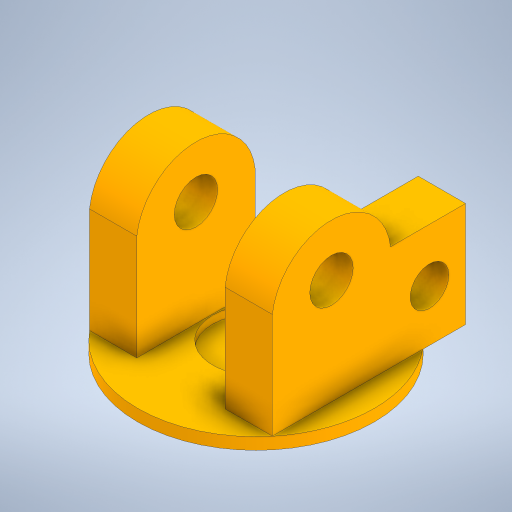
# Autodesk Inventor part: base2
Saved by Autodesk Inventor 2024 (Build 280153000, 153)
## iProperties
Created: 2024-04-28
Part Number: base2
Material: Generic
Document SubType Name: Modeling
Designer: samue
Density: 1 g/cm^3
Appearance: Default
Author: samue
## iProperties of the stored document base2_3DPrint.ipt
Created: 2024-04-28
Part Number: base2_3DPrint
Material: Generic
Document SubType Name: Modeling
Designer: samue
Density: 1 g/cm^3
Appearance: Default
Author: samue
Autodesk Inventor part; units mm, degrees
ref_plane "YZ Plane" through (0, 0, 0) normal (1, 0, 0) x (0, 1, 0)
ref_plane "XZ Plane" through (0, 0, 0) normal (0, 1, 0) x (-1, 0, 0)
ref_plane "XY Plane" through (0, 0, 0) normal (0, 0, 1) x (1, 0, 0)
sketch "Sketch1" plane through (0, 0, 0) normal (0, 1, 0) x (-1, 0, 0)
  circle A0 centre (0, 0) radius 30
  dimension "d0" = 60
  constraints: 1 centre point, 1 coincident
  measures "d0" diameter of A0
extrude "Extrusion1" add sketch "Sketch1" along normal blind 3
sketch "Sketch2" plane through (0, 3, 0) normal (0, 1, 0) x (1, 0, 0)
  circle A0 centre (0, 0) radius 5
  dimension "d3" = 10
  constraints: 1 centre point, 1 coincident
  measures "d3" diameter of A0
extrude "Extrusion2" cut sketch "Sketch2" against normal blind 4
sketch "Sketch3" plane through (0, 3, 0) normal (0, 1, 0) x (1, 0, 0)
  circle A0 centre (0, 0) radius 5 projected
  circle A1 centre (0, 0) radius 11
  dimension "d6" = 22
  constraints: 1 centre point, 1 coincident
  measures "d6" diameter of A1
extrude "Extrusion3" cut sketch "Sketch3" against normal blind 2
sketch "Sketch4" plane through (0, 3, 0) normal (0, 1, 0) x (1, 0, 0)
  line L0 (-23.2158, -19.0158) -> (-11.2158, -19.0158)
  line L1 (-11.2158, -19.0158) -> (-11.2158, 10.9842)
  line L2 (-11.2158, 10.9842) -> (-23.2158, 10.9842)
  line L3 (-23.2158, 10.9842) -> (-23.2158, -19.0158)
  line L4 (-0.0289, -32.9889) -> (-0.0289, 43.4959) construction
  line L5 (23.1581, -19.0158) -> (11.1581, -19.0158)
  line L6 (11.1581, -19.0158) -> (11.1581, 10.9842)
  line L7 (11.1581, 10.9842) -> (23.1581, 10.9842)
  line L8 (23.1581, 10.9842) -> (23.1581, -19.0158)
  point P0 (0, -4.0158)
  point P1 (-23.2158, -4.0158)
  point P2 (23.2158, 0)
  dimension "d9" = 12
  dimension "d10" = 30
  constraints: 16 end point, 4 symmetric about line, 2 parallel, 1 horizontal, 1 horizontal alignment, 1 midpoint, 1 perpendicular, 1 vertical, 3 other
  measures "d9" distance of L2.end L1.end
  measures "d10" distance of L1.end L0.end
extrude "Extrusion4" add sketch "Sketch4" along normal blind 40
sketch "Sketch5" plane through (23.1581, 3, 19.0158) normal (1, 0, 0) x (0, 0, -1)
  line L0 (30, 0) -> (30, 40) projected
  line L1 (0, 0) -> (0, 40) projected
  arc A0 (30, 26.6004) -> (0, 26.7351) centre (14.9918, 24.8495) ccw
  line L2 (0, 26.7351) -> (0, 40)
  line L3 (30, 40) -> (0, 40) projected
  line L4 (30, 40) -> (30, 26.6004)
  point P0 (19.0158, -3)
  constraints: 4 end point, 2 point on circle, 2 point on line, 1 centre point, 1 collinear, 1 perpendicular
extrude "Extrusion5" cut sketch "Sketch5" against normal blind 74.5
sketch "Sketch6" plane through (23.1581, 3, 19.0158) normal (1, 0, 0) x (0, 0, -1)
  circle A0 centre (15, 26.7283) radius 5.5
  point P0 (19.0158, -3)
  dimension "d15" = 11
  constraints: 1 centre point
  measures "d15" diameter of A0
extrude "Extrusion6" cut sketch "Sketch6" against normal blind 74.5
sketch "Sketch7" plane through (23.1581, 3, 19.0158) normal (1, 0, 0) x (0, 0, -1)
  line L0 (30, 0) -> (30, 26.6004) projected
  line L1 (30, 26.6004) -> (49.0158, 26.6004)
  line L2 (49.0158, 0) -> (-10.9842, 0) projected
  line L3 (49.0158, 26.6004) -> (49.0158, 0)
  point P0 (19.0158, -3)
  point P1 (0, 0)
  point P2 (0.0152, 0)
  constraints: 4 end point, 1 horizontal, 1 vertical
extrude "Extrusion7" add sketch "Sketch7" against normal blind 12
sketch "Sketch8" plane through (23.1581, 3, 19.0158) normal (1, 0, 0) x (0, 0, -1)
  circle A0 centre (39.8603, 13.0279) radius 4.9
  point P0 (19.0158, -3)
  dimension "d20" = 9.8
  constraints: 1 centre point
  measures "d20" diameter of A0
extrude "Extrusion8" cut sketch "Sketch8" against normal blind 12
body "Solid1"
